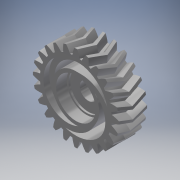
# Autodesk Inventor part: Stirnzahnrad1
Saved by Autodesk Inventor 2019.1 (Build 231200000, 200)
## iProperties
Created: 2019-01-01
Part Number: Stirnzahnrad1
Material: Steel
Document SubType Name: Modeling
Designer: JochenAlt
Categories: <?xml version="1.0" encoding="UTF-16"?> <MemberInstance><Categories><FamilyTemplate><FamilyTemplateParameter ValueType="xs:double" Id="1" ObjectReferenceKey="da_z" ObjectType="kUserParameterObject"/><FamilyTemplateParameter ValueType="xs:double" Id="2" ObjectReferenceKey="da_b" ObjectType="kUserParameterObject"/><FamilyTemplateParameter ValueType="xs:double" Id="3" ObjectReferenceKey="da_beta" ObjectType="kUserParameterObject"/><FamilyTemplateParameter ValueType="xs:double" Id="4" ObjectReferenceKey="da_da" ObjectType="kUserParameterObject"/><FamilyTemplateParameter ValueType="xs:double" Id="5" ObjectReferenceKey="da_aw" ObjectType="kUserParameterObject"/><FamilyTemplateParameter ValueType="xs:string" Id="6" ObjectReferenceKey="EAIAABAAAACIAQAAAAAAAIAAAAAAAAAA" ObjectType="83910656" SubObjectId="SurfaceGeometry"/></FamilyTemplate><ParamToTemplateMap><ParamToTemplate CategoryParameter="//CategoryParameter[@InternalName='046C89C9-8512-4d59-83FE-43B91F4F132A']" TemplateParameter="1"/><ParamToTemplate CategoryParameter="//CategoryParameter[@InternalName='2552DF32-E462-4b46-AEBF-C6C7768E72AC']" TemplateParameter="2"/><ParamToTemplate CategoryParameter="//CategoryParameter[@InternalName='C9EE641D-15FC-4fae-A226-E94C4372FDD7']" TemplateParameter="3"/><ParamToTemplate><ParamToTemplate CategoryParameter="//CategoryParameter[@InternalName='00B6519A-459B-49c7-AD84-2E56D39A5744']" ConstantValue="-0.200000"/></ParamToTemplate><ParamToTemplate><ParamToTemplate CategoryParameter="//CategoryParameter[@InternalName='04B31F0E-C7A6-4894-AA32-9629BEFACF47']" ConstantValue="1.000000"/></ParamToTemplate><ParamToTemplate><ParamToTemplate CategoryParameter="//CategoryParameter[@InternalName='43CBEC2E-7847-49e7-A936-2F7889FCB2D9']" ConstantValue="0.250000"/></ParamToTemplate><ParamToTemplate><ParamToTemplate CategoryParameter="//CategoryParameter[@InternalName='B1EFC894-105D-4ebd-86BF-FA20ED196853']" ConstantValue="0.350000"/></ParamToTemplate><ParamToTemplate><ParamToTemplate CategoryParameter="//CategoryParameter[@InternalName='51175063-3D10-4879-93E8-6246FE8B403D']" ConstantValue="2060000000.000000"/></ParamToTemplate><ParamToTemplate><ParamToTemplate CategoryParameter="//CategoryParameter[@InternalName='A3A52E27-4454-46a9-B0BD-C932399B70AF']" ConstantValue="0.300000"/></ParamToTemplate><ParamToTemplate><ParamToTemplate CategoryParameter="//CategoryParameter[@InternalName='91B76062-C214-41d9-B1B9-14D2AB99603D']" ConstantValue="0.090000"/></ParamToTemplate><ParamToTemplate><ParamToTemplate CategoryParameter="//CategoryParameter[@InternalName='374E806E-8B8A-4dda-A9AA-1039D6500AD2']" ConstantValue="11.111111"/></ParamToTemplate><ParamToTemplate><ParamToTemplate CategoryParameter="//CategoryParameter[@InternalName='2D373A89-B862-43d6-8D0B-0CBF12AB9F6C']" ConstantValue="0.349066"/></ParamToTemplate><ParamToTemplate CategoryParameter="//CategoryParameter[@InternalName='37777632-D6A2-4fac-9D53-DB8ACD95C989']" TemplateParameter="4"/><ParamToTemplate CategoryParameter="//CategoryParameter[@InternalName='FD1017F1-B727-4f7e-9707-0F86F1FF9423']" TemplateParameter="5"/><ParamToTemplate><ParamToTemplate CategoryParameter="//CategoryParameter[@InternalName='9E1B4470-B2D3-4ff1-B813-535BB4CDF51A']" ConstantValue="3520000.000000"/></ParamToTemplate><ParamToTemplate><ParamToTemplate CategoryParameter="//CategoryParameter[@InternalName='F8452263-BFF6-458c-9FB1-07C4B99E95CD']" ConstantValue="11400000.000000"/></ParamToTemplate><ParamToTemplate><ParamToTemplate CategoryParameter="//CategoryParameter[@InternalName='3E3BB259-FD49-497f-8171-6EBC954A3479']" ConstantValue="2.000000"/></ParamToTemplate><ParamToTemplate CategoryParameter="//CategoryParameter[@InternalName='27C3BAF2-7550-4e4b-AE2C-0DB134B7D9B7']" TemplateParameter="6"/></ParamToTemplateMap><Category DisplayName="Gear" InternalName="DC85795E-93AB-48d5-8EEE-5A27447B64BD" Mnemonic="Gear"><CategoryParameter DisplayName="z" InternalName="046C89C9-8512-4d59-83FE-43B91F4F132A" Mnemonic="z"/><CategoryParameter DisplayName="b" InternalName="2552DF32-E462-4b46-AEBF-C6C7768E72AC" Mnemonic="b"/><CategoryParameter DisplayName="||b|" InternalName="C9EE641D-15FC-4fae-A226-E94C4372FDD7" Mnemonic="beta"/><CategoryParameter DisplayName="x" InternalName="00B6519A-459B-49c7-AD84-2E56D39A5744" Mnemonic="x"/><CategoryParameter DisplayName="a*" InternalName="04B31F0E-C7A6-4894-AA32-9629BEFACF47" Mnemonic="a"/><CategoryParameter DisplayName="c*" InternalName="43CBEC2E-7847-49e7-A936-2F7889FCB2D9" Mnemonic="c"/><CategoryParameter DisplayName="r|.f|*" InternalName="B1EFC894-105D-4ebd-86BF-FA20ED196853" Mnemonic="rf"/><CategoryParameter DisplayName="E" InternalName="51175063-3D10-4879-93E8-6246FE8B403D" Mnemonic="E"/><CategoryParameter DisplayName="||m|" InternalName="A3A52E27-4454-46a9-B0BD-C932399B70AF" Mnemonic="mi"/><Category DisplayName="SpurGear" InternalName="26C5A22E-A91E-4dfd-A3B3-23CCAFAE1764" Mnemonic="SpurGear"><CategoryParameter DisplayName="m" InternalName="91B76062-C214-41d9-B1B9-14D2AB99603D" Mnemonic="m"/><CategoryParameter DisplayName="P" InternalName="374E806E-8B8A-4dda-A9AA-1039D6500AD2" Mnemonic="PP"/><CategoryParameter DisplayName="||a|" InternalName="2D373A89-B862-43d6-8D0B-0CBF12AB9F6C" Mnemonic="alpha"/><CategoryParameter DisplayName="d|.a|" InternalName="37777632-D6A2-4fac-9D53-DB8ACD95C989" Mnemonic="da"/><CategoryParameter DisplayName="a|.w|" InternalName="FD1017F1-B727-4f7e-9707-0F86F1FF9423" Mnemonic="aw"/><CategoryParameter DisplayName="||s||.Flim|" InternalName="9E1B4470-B2D3-4ff1-B813-535BB4CDF51A" Mnemonic="sFlim"/><CategoryParameter DisplayName="||s||.Hlim|" InternalName="F8452263-BFF6-458c-9FB1-07C4B99E95CD" Mnemonic="sHlim"/><CategoryParameter DisplayName="Typ" InternalName="3E3BB259-FD49-497f-8171-6EBC954A3479" Mnemonic="type"/><CategoryParameter DisplayName="PitchDiameter" InternalName="27C3BAF2-7550-4e4b-AE2C-0DB134B7D9B7" Mnemonic="IDS_PITCHDIAM"/></Category></Category></Categories></MemberInstance>
Density: 1 g/cm^3
Appearance: Steel
CustomPartVersion: 1
Author: JochenAlt
Autodesk Inventor part; units mm, degrees
ref_plane "YZ Plane" through (0, 0, 0) normal (1, 0, 0) x (0, 1, 0)
ref_plane "XZ Plane" through (0, 0, 0) normal (0, 1, 0) x (-1, 0, 0)
ref_plane "XY Plane" through (0, 0, 0) normal (0, 0, 1) x (1, 0, 0)
sketch "Sketch1" plane through (0, 0, 0) normal (0, 0, 1) x (1, 0, 0)
  circle A0 centre (0, 0) radius 12.1809
  dimension "d0" = 24.3618
  constraints: 1 centre point
  measures "d0" diameter of A0
extrude "Extrusion1" add sketch "Sketch1" along normal blind 4
ref_plane "Work Plane2" through (0, 0, 2) normal (0, 0, 1) x (1, 0, 0)
sketch "Sketch2" plane through (0, 0, 0) normal (0, 0, -1) x (-1, 0, 0)
  circle A0 centre (0, 0) radius 12.1809 projected
  circle A1 centre (0, 0) radius 11.2316
  dimension "d3" = 22.4632
  constraints: 1 centre point, 1 coincident
  measures "d3" diameter of A1
surface extrude "Flankendurchmesser" sketch "Sketch2" against normal through all shown no curves A1
ref_plane "Work Plane8" through (0, 0, 0) normal (0.9914449, 0.1305262, 0) x (0, 0, 1)
ref_plane "Work Plane9" through (0, 0, 0) normal (1, 0, 0) x (0, 1, 0)
spur gear teeth "Stirnzahnrad" teeth 24 pitch diameter 22.9862 tip diameter 24.3618 root diameter 20.3762 face width 4 helix angle 20 hand left start plane through (0, 0, 0) normal (0, 0, -1) x (-1, 0, 0)
sketch "Skizze3" plane through (0, 0, 4) normal (0, 0, 1) x (1, 0, 0)
  circle A0 centre (0, 0) radius 2.4
  circle A1 centre (0, 0) radius 5.6
  circle A2 centre (0, 0) radius 5.1
  circle A3 centre (0, 0) radius 10.1881 construction
  arc A4 (-5.6699, -3.3782) -> (0.6484, -6.5681) centre (0, 0) ccw
  arc A5 (-6.2254, 6.7576) -> (-9.09, -1.3393) centre (0, 0) ccw
  arc A6 (5.6699, -3.3782) -> (5.3106, 3.9189) centre (0, 0) ccw
  arc A7 (0, 6.6) -> (-6.0848, 2.5563) centre (0, 0) ccw
  arc A8 (-2.9795, -8.6916) -> (5.8033, -7.1234) centre (0, 0) ccw
  line L0 (0, 0) -> (0, 9.1881) construction
  line L1 (0, 0) -> (-7.8933, -4.7029) construction
  line L2 (0, 0) -> (7.8933, -4.7029) construction
  arc A9 (5.8033, -7.1234) -> (8.9918, 1.8892) centre (0, 0) ccw construction
  arc A10 (3.1492, 8.6316) -> (-6.2254, 6.7576) centre (0, 0) ccw construction
  arc A11 (-9.09, -1.3393) -> (-2.9795, -8.6916) centre (0, 0) ccw construction
  line L3 (1.4545, 6.6) -> (0, 6.6) construction
  arc A12 (5.8033, -7.1234) -> (5.3106, 3.9189) centre (1.4545, -1.7853) ccw
  line L4 (1.4545, 5.1) -> (7.6427, 5.1) construction
  line L5 (0, 6.6) -> (1.4545, 6.6)
  arc A13 (8.9918, 1.8892) -> (3.1492, 8.6316) centre (0, 0) ccw
  arc A14 (8.9918, 1.8892) -> (1.4545, 6.6) centre (1.4545, -1.7853) ccw
  line L6 (5.6699, -3.3782) -> (4.9254, -4.6277)
  arc A15 (-2.9795, -8.6916) -> (4.9254, -4.6277) centre (-2.2782, -0.3357) ccw
  arc A16 (-9.09, -1.3393) -> (0.6484, -6.5681) centre (-2.2782, -0.3357) ccw
  arc A17 (3.1492, 8.6316) -> (-6.0848, 2.5563) centre (0.7893, 2.1633) ccw
  line L7 (-5.6699, -3.3782) -> (-6.4144, -2.1287)
  arc A18 (-6.2254, 6.7576) -> (-6.4144, -2.1287) centre (0.7893, 2.1633) ccw
  arc A19 (0.6484, -6.5681) -> (5.5616, -3.3137) centre (-0.1562, -0.0173) ccw construction
  arc A20 (-6.0848, 2.5563) -> (-5.6699, -3.3782) centre (0, 0) ccw construction
  arc A21 (5.3106, 3.9189) -> (0, 6.6) centre (0, 0) ccw construction
  point P0 (0.2903, 10.184)
  dimension "d49" = 4.8
  dimension "d50" = 11.2
  dimension "d52" = 0.5
  dimension "d62" = 4.7029
  dimension "d63" = 1
  dimension "d64" = 1
  dimension "d70" = 1.5
  constraints: 46 point on circle, 21 centre point, 16 end point, 11 tangent, 10 coincident, 10 equal radius, 5 point on line, 2 concentric, 2 equal length, 1 parallel, 1 vertical, 4 other
  measures "d49" diameter of A0
  measures "d50" diameter of A1
  measures "d52" radial gap between concentric circles of A1 A2
  measures "d62" vertical distance of L0.start L1.end
  measures "d63" radial gap between concentric circles of A6 A1
  measures "d70" distance between parallel lines of L4 L3
extrude "Extrusion5" cut sketch "Skizze3" against normal through all contours A4 A16 A5 A18 L7 | A6 A12 A8 A15 L6 | A7 A17 A13 A14 L5
mirror "Spiegeln1" about plane through (0, 0, 4) normal (0, 0, 1)
extrude "Extrusion2" cut sketch "Skizze3" against normal blind 3 from surface at 4 contours A0 | A1 | A2
extrude "Extrusion3" cut sketch "Skizze3" against normal blind 0.5 from surface at 1 contours A2
extrude "Extrusion4" cut sketch "Skizze3" along normal through all both and the other way through all contours A0
equation "\"d0\" = da_da"
equation "\"d1\" = da_b"
equation "\"d3\" = da_dw"
equation "\"d16\" = da_aw"
equation "\"d43\" = da_aw"
equation "\"d46\" = da_aw"
equation "\"da_da\" = 24.361758"
equation "\"da_b\" = 4"
equation "\"da_dw\" = 22.463252"
equation "\"da_aw\" = 16.847439"
body "Solid1"
body "Srf1"
